Autodesk Fusion 360 part; units mm, degrees
(part 3 of 6)
sketch "top plate" plane through (0, 0, 0) normal (0, 1, 0) x (1, 0, 0)
  line L0 (103.8578, -14.9931) -> (9.2428, -14.9931)
  line L1 (9.2428, -110.3136) -> (21.2428, -111.7953)
  line L2 (21.2428, -111.7953) -> (66.9572, -117.4397)
  line L3 (66.9572, -117.4397) -> (84.9842, -117.4397)
  line L4 (123.6486, -112.6772) -> (84.9842, -117.4397)
  arc A0 (138.7122, -103.2228) -> (142.7339, -99.2011) centre (138.7122, -99.2011) ccw
  arc A1 (146.7556, -80.8214) -> (142.7339, -84.843) centre (146.7556, -84.843) ccw
  arc A2 (146.7556, -80.8214) -> (146.7556, -72.7781) centre (146.7556, -76.7997) ccw
  arc A3 (142.7339, -68.7564) -> (146.7556, -72.7781) centre (146.7556, -68.7564) ccw
  arc A4 (146.8111, -48.4919) -> (142.7339, -52.5692) centre (146.8111, -52.5692) ccw
  arc A5 (157.6917, -48.4919) -> (157.6917, -40.3375) centre (157.6917, -44.4147) ccw
  arc A6 (150.7772, -36.2632) -> (154.8573, -40.3375) centre (154.8544, -36.2603) ccw
  line L5 (142.6281, 7.5847) -> (103.8578, -14.9931)
  line L6 (142.6281, 7.5847) -> (161.7839, -25.5411)
  line L7 (132.0216, -103.2228) -> (138.7122, -103.2228)
  line L8 (142.7339, -99.2011) -> (142.7339, -84.843)
  line L9 (142.7339, -52.5692) -> (142.7339, -68.7564)
  line L10 (146.8111, -48.4919) -> (157.6917, -48.4919)
  line L11 (157.6917, -40.3375) -> (154.8573, -40.3375)
  line L12 (9.2428, -110.3136) -> (9.2428, -14.9931)
  line L13 (11.8031, -107.7533) -> (25.8031, -107.7533)
  line L14 (25.8031, -107.7533) -> (25.8031, -93.7533)
  line L15 (25.8031, -93.7533) -> (11.8031, -93.7533)
  line L16 (11.8031, -93.7533) -> (11.8031, -107.7533)
  line L17 (30.8531, -107.7533) -> (44.8531, -107.7533)
  line L18 (44.8531, -107.7533) -> (44.8531, -93.7533)
  line L19 (44.8531, -93.7533) -> (30.8531, -93.7533)
  line L20 (30.8531, -93.7533) -> (30.8531, -107.7533)
  line L21 (49.9031, -112.5158) -> (63.9031, -112.5158)
  line L22 (63.9031, -112.5158) -> (63.9031, -98.5158)
  line L23 (63.9031, -98.5158) -> (49.9031, -98.5158)
  line L24 (49.9031, -98.5158) -> (49.9031, -112.5158)
  line L25 (88.0031, -112.5158) -> (102.0031, -112.5158)
  line L26 (102.0031, -112.5158) -> (102.0031, -98.5158)
  line L27 (102.0031, -98.5158) -> (88.0031, -98.5158)
  line L28 (107.0531, -110.1169) -> (121.0531, -110.1169)
  line L29 (121.0531, -110.1169) -> (121.0531, -96.1169)
  line L30 (121.0531, -96.1169) -> (107.0531, -96.1169)
  line L31 (107.0531, -96.1169) -> (107.0531, -110.1169)
  line L32 (140.1031, -100.5919) -> (126.1031, -100.5919)
  line L33 (126.1031, -100.5919) -> (126.1031, -86.5919)
  line L34 (126.1031, -86.5919) -> (140.1031, -86.5919)
  line L35 (140.1031, -86.5919) -> (140.1031, -100.5919)
  line L36 (126.1031, -81.5419) -> (140.1031, -81.5419)
  line L37 (140.1031, -81.5419) -> (140.1031, -67.5419)
  line L38 (140.1031, -67.5419) -> (126.1031, -67.5419)
  line L39 (126.1031, -67.5419) -> (126.1031, -81.5419)
  line L40 (126.1031, -62.4919) -> (140.1031, -62.4919)
  line L41 (140.1031, -62.4919) -> (140.1031, -48.4919)
  line L42 (140.1031, -48.4919) -> (126.1031, -48.4919)
  line L43 (126.1031, -48.4919) -> (126.1031, -62.4919)
  line L44 (49.9031, -93.4658) -> (63.9031, -93.4658)
  line L45 (63.9031, -93.4658) -> (63.9031, -79.4658)
  line L46 (63.9031, -79.4658) -> (49.9031, -79.4658)
  line L47 (49.9031, -79.4658) -> (49.9031, -93.4658)
  line L48 (49.9031, -74.4158) -> (63.9031, -74.4158)
  line L49 (63.9031, -74.4158) -> (63.9031, -60.4158)
  line L50 (63.9031, -60.4158) -> (49.9031, -60.4158)
  line L51 (49.9031, -60.4158) -> (49.9031, -74.4158)
  line L52 (49.9031, -55.3658) -> (63.9031, -55.3658)
  line L53 (63.9031, -55.3658) -> (63.9031, -41.3658)
  line L54 (63.9031, -41.3658) -> (49.9031, -41.3658)
  line L55 (49.9031, -41.3658) -> (49.9031, -55.3658)
  line L56 (30.8531, -88.7033) -> (44.8531, -88.7033)
  line L57 (44.8531, -88.7033) -> (44.8531, -74.7033)
  line L58 (44.8531, -74.7033) -> (30.8531, -74.7033)
  line L59 (30.8531, -74.7033) -> (30.8531, -88.7033)
  line L60 (30.8531, -69.6533) -> (44.8531, -69.6533)
  line L61 (44.8531, -69.6533) -> (44.8531, -55.6533)
  line L62 (44.8531, -55.6533) -> (30.8531, -55.6533)
  line L63 (30.8531, -55.6533) -> (30.8531, -69.6533)
  line L64 (11.8031, -88.7033) -> (25.8031, -88.7033)
  line L65 (25.8031, -88.7033) -> (25.8031, -74.7033)
  line L66 (25.8031, -74.7033) -> (11.8031, -74.7033)
  line L67 (11.8031, -74.7033) -> (11.8031, -88.7033)
  line L68 (11.8031, -69.6533) -> (25.8031, -69.6533)
  line L69 (25.8031, -69.6533) -> (25.8031, -55.6533)
  line L70 (25.8031, -55.6533) -> (11.8031, -55.6533)
  line L71 (11.8031, -55.6533) -> (11.8031, -69.6533)
  line L72 (11.8031, -50.6033) -> (25.8031, -50.6033)
  line L73 (25.8031, -50.6033) -> (25.8031, -36.6033)
  line L74 (25.8031, -36.6033) -> (11.8031, -36.6033)
  line L75 (11.8031, -36.6033) -> (11.8031, -50.6033)
  line L76 (30.8531, -50.6033) -> (44.8531, -50.6033)
  line L77 (44.8531, -50.6033) -> (44.8531, -36.6033)
  line L78 (44.8531, -36.6033) -> (30.8531, -36.6033)
  line L79 (30.8531, -36.6033) -> (30.8531, -50.6033)
  line L80 (11.8031, -31.5533) -> (25.8031, -31.5533)
  line L81 (25.8031, -31.5533) -> (25.8031, -17.5533)
  line L82 (25.8031, -17.5533) -> (11.8031, -17.5533)
  line L83 (11.8031, -17.5533) -> (11.8031, -31.5533)
  line L84 (30.8531, -31.5533) -> (44.8531, -31.5533)
  line L85 (44.8531, -31.5533) -> (44.8531, -17.5533)
  line L86 (44.8531, -17.5533) -> (30.8531, -17.5533)
  line L87 (30.8531, -17.5533) -> (30.8531, -31.5533)
  line L88 (49.9031, -36.3158) -> (63.9031, -36.3158)
  line L89 (63.9031, -36.3158) -> (63.9031, -22.3158)
  line L90 (63.9031, -22.3158) -> (49.9031, -22.3158)
  line L91 (49.9031, -22.3158) -> (49.9031, -36.3158)
  line L92 (68.9531, -114.8794) -> (82.9531, -114.8794)
  line L93 (82.9531, -114.8794) -> (82.9531, -100.8794)
  line L94 (82.9531, -100.8794) -> (68.9531, -100.8794)
  line L95 (68.9531, -100.8794) -> (68.9531, -114.8794)
  line L96 (68.9531, -95.8294) -> (82.9531, -95.8294)
  line L97 (82.9531, -95.8294) -> (82.9531, -81.8294)
  line L98 (82.9531, -81.8294) -> (68.9531, -81.8294)
  line L99 (68.9531, -81.8294) -> (68.9531, -95.8294)
  line L100 (68.9531, -76.7794) -> (82.9531, -76.7794)
  line L101 (82.9531, -76.7794) -> (82.9531, -62.7794)
  line L102 (82.9531, -62.7794) -> (68.9531, -62.7794)
  line L103 (68.9531, -62.7794) -> (68.9531, -76.7794)
  line L104 (68.9531, -57.7294) -> (82.9531, -57.7294)
  line L105 (82.9531, -57.7294) -> (82.9531, -43.7294)
  line L106 (82.9531, -43.7294) -> (68.9531, -43.7294)
  line L107 (68.9531, -43.7294) -> (68.9531, -57.7294)
  line L108 (76.5731, -36.3158) -> (90.5731, -36.3158)
  line L109 (90.5731, -36.3158) -> (90.5731, -22.3158)
  line L110 (90.5731, -22.3158) -> (76.5731, -22.3158)
  line L111 (76.5731, -22.3158) -> (76.5731, -36.3158)
  line L112 (88.0031, -74.4158) -> (102.0031, -74.4158)
  line L113 (102.0031, -74.4158) -> (102.0031, -60.4158)
  line L114 (102.0031, -60.4158) -> (88.0031, -60.4158)
  line L115 (88.0031, -60.4158) -> (88.0031, -74.4158)
  line L116 (107.0531, -77.0669) -> (121.0531, -77.0669)
  line L117 (121.0531, -77.0669) -> (121.0531, -91.0669)
  line L118 (121.0531, -91.0669) -> (107.0531, -91.0669)
  line L119 (107.0531, -91.0669) -> (107.0531, -77.0669)
  line L120 (88.0031, -93.4658) -> (102.0031, -93.4658)
  line L121 (102.0031, -93.4658) -> (102.0031, -79.4658)
  line L122 (102.0031, -79.4658) -> (88.0031, -79.4658)
  line L123 (88.0031, -79.4658) -> (88.0031, -93.4658)
  line L124 (107.0531, -72.0169) -> (121.0531, -72.0169)
  line L125 (121.0531, -72.0169) -> (121.0531, -58.0169)
  line L126 (121.0531, -58.0169) -> (107.0531, -58.0169)
  line L127 (107.0531, -58.0169) -> (107.0531, -72.0169)
  line L128 (107.0531, -52.9669) -> (121.0531, -52.9669)
  line L129 (121.0531, -52.9669) -> (121.0531, -38.9669)
  line L130 (121.0531, -38.9669) -> (107.0531, -38.9669)
  line L131 (107.0531, -38.9669) -> (107.0531, -52.9669)
  line L132 (88.0031, -55.3658) -> (102.0031, -55.3658)
  line L133 (102.0031, -55.3658) -> (102.0031, -41.3658)
  line L134 (102.0031, -41.3658) -> (88.0031, -41.3658)
  line L135 (88.0031, -41.3658) -> (88.0031, -55.3658)
  line L136 (88.0031, -112.5158) -> (88.0031, -98.5158)
  circle A7 centre (28.3281, -91.2283) radius 1.1
  circle A8 centre (18.8031, -34.0783) radius 1.1
  circle A9 centre (71.0494, -18.8031) radius 1.1
  circle A10 centre (95.25, -34.2547) radius 1.1
  circle A11 centre (115.7464, -33.7256) radius 1.1
  circle A12 centre (146.7556, -76.7997) radius 1.1
  circle A13 centre (157.6917, -44.4147) radius 1.1
  circle A14 centre (146.7556, -37.8883) radius 1.1
  circle A15 centre (123.5781, -102.5878) radius 1.1
  circle A16 centre (66.4281, -78.105) radius 1.1
  circle A17 centre (130.9158, -10.2658) radius 1.1
  line L137 (104.7731, -17.2287) -> (111.7731, -29.353)
  line L138 (111.7731, -29.353) -> (123.8975, -22.353)
  line L139 (123.8975, -22.353) -> (116.8975, -10.2287)
  line L140 (116.8975, -10.2287) -> (104.7731, -17.2287)
  line L141 (139.0984, -19.4159) -> (146.0984, -31.5402)
  line L142 (146.0984, -31.5402) -> (158.2227, -24.5402)
  line L143 (158.2227, -24.5402) -> (151.2227, -12.4159)
  line L144 (151.2227, -12.4159) -> (139.0984, -19.4159)
  line L145 (161.7839, -25.5411) -> (150.0604, -32.3205)
  line L146 (154.8544, -36.2603) -> (154.8544, -34.2581)
  line L147 (150.7772, -36.2632) -> (150.7772, -32.2)
  line L148 (154.8544, -34.2581) -> (152.8134, -30.7285)
  arc A18 (152.8134, -30.7285) -> (150.7772, -34.2581) centre (154.8544, -34.2581) ccw
  line L149 (122.5884, -28.9762) -> (129.5884, -41.1005)
  line L150 (129.5884, -41.1005) -> (141.7127, -34.1005)
  line L151 (141.7127, -34.1005) -> (134.7127, -21.9762)
  line L152 (134.7127, -21.9762) -> (122.5884, -28.9762)
  line L153 (129.5734, -2.9059) -> (136.5734, -15.0302)
  line L154 (136.5734, -15.0302) -> (148.6977, -8.0302)
  line L155 (148.6977, -8.0302) -> (141.6977, 4.0941)
  line L156 (141.6977, 4.0941) -> (129.5734, -2.9059)
  line L157 (123.6486, -112.6772) -> (123.6486, -108.4548)
  line L158 (123.6486, -108.4548) -> (127.6703, -108.4548)
  arc A19 (126.6957, -104.553) -> (123.6486, -108.4548) centre (127.6703, -108.4548) ccw
  line L159 (132.0216, -103.2228) -> (126.6957, -104.553)
  line L160 (127.6703, -108.4548) -> (126.6957, -104.553)
  line L161 (161.7839, -103.1522) -> (123.6486, -112.6772)
  line L162 (103.943, -25.7908) -> (124.7276, -13.7908)
  line L163 (98.3098, -21.884) -> (104.5098, -32.6227)
  line L164 (104.5098, -32.6227) -> (109.5761, -29.6977)
  line L165 (109.5761, -29.6977) -> (103.3761, -18.959)
  line L166 (103.3761, -18.959) -> (98.3098, -21.884)
  line L167 (124.1607, -6.959) -> (130.3607, -17.6977)
  line L168 (130.3607, -17.6977) -> (125.2945, -20.6227)
  line L169 (125.2945, -20.6227) -> (119.0945, -9.884)
  line L170 (119.0945, -9.884) -> (124.1607, -6.959)
  line L171 (107.9761, -26.9264) -> (109.7731, -25.8889)
  line L172 (104.9761, -21.7303) -> (106.7731, -20.6928)
  line L173 (121.8975, -18.8889) -> (123.6945, -17.8514)
  line L174 (118.8975, -13.6928) -> (120.6945, -12.6553)
  line L175 (131.5417, -103.3426) -> (132.5162, -107.2444)
  line L176 (132.5162, -103.2228) -> (132.5162, -107.2444)
  arc A20 (132.5162, -103.2228) -> (131.5417, -103.3426) centre (132.5162, -107.2444) ccw
  point P0 (132.0216, -103.2228)
  point P1 (18.8031, -100.7533)
  point P2 (37.8531, -100.7533)
  point P3 (37.8531, -81.7033)
  point P4 (28.3281, -91.2283)
  point P5 (18.8031, -81.7033)
  point P6 (56.9031, -105.5158)
  point P7 (56.9031, -86.4658)
  point P8 (18.8031, -62.6533)
  point P9 (37.8531, -62.6533)
  point P10 (56.9031, -67.4158)
  point P11 (56.9031, -48.3658)
  point P12 (37.8531, -43.6033)
  point P13 (18.8031, -43.6033)
  point P14 (18.8031, -24.5533)
  point P15 (18.8031, -34.0783)
  point P16 (37.8531, -24.5533)
  point P17 (56.9031, -29.3158)
  point P18 (71.0494, -18.8031)
  point P19 (83.5731, -29.3158)
  point P20 (95.25, -34.2547)
  point P21 (115.7464, -33.7256)
  point P22 (114.3353, -19.7908)
  point P23 (132.1506, -31.5383)
  point P24 (130.9158, -10.2658)
  point P25 (139.1356, -5.4681)
  point P26 (148.6606, -21.9781)
  point P27 (146.7556, -37.8883)
  point P28 (157.6917, -44.4147)
  point P29 (114.0531, -45.9669)
  point P30 (133.1031, -55.4919)
  point P31 (114.0531, -65.0169)
  point P32 (95.0031, -48.3658)
  point P33 (95.0031, -67.4158)
  point P34 (133.1031, -74.5419)
  point P35 (146.7556, -76.7997)
  point P36 (133.1031, -93.5919)
  point P37 (123.5781, -102.5878)
  point P38 (114.0531, -103.1169)
  point P39 (114.0531, -84.0669)
  point P40 (95.0031, -86.4658)
  point P41 (95.0031, -105.5158)
  point P42 (66.4281, -78.105)
  point P43 (75.9531, -107.8794)
  point P44 (75.9531, -88.8294)
  point P45 (75.9531, -69.7794)
  point P46 (75.9531, -50.7294)
  dimension "d126" = 14
  dimension "d127" = 14
  dimension "d128" = 7
  dimension "d129" = 7
  dimension "d130" = 14
  dimension "d131" = 14
  dimension "d132" = 14
  dimension "d133" = 14
  dimension "d134" = 14
  dimension "d135" = 14
  dimension "d136" = 14
  dimension "d137" = 14
  dimension "d138" = 14
  dimension "d139" = 14
  dimension "d140" = 14
  dimension "d141" = 14
  dimension "d142" = 14
  dimension "d143" = 14
  dimension "d144" = 14
  dimension "d145" = 14
  dimension "d146" = 14
  dimension "d147" = 14
  dimension "d148" = 14
  dimension "d149" = 14
  dimension "d150" = 14
  dimension "d151" = 14
  dimension "d152" = 14
  dimension "d153" = 14
  dimension "d154" = 14
  dimension "d155" = 14
  dimension "d156" = 14
  dimension "d157" = 14
  dimension "d158" = 14
  dimension "d159" = 14
  dimension "d160" = 14
  dimension "d161" = 14
  dimension "d162" = 14
  dimension "d163" = 14
  dimension "d164" = 14
  dimension "d165" = 14
  dimension "d166" = 14
  dimension "d167" = 14
  dimension "d168" = 14
  dimension "d170" = 14
  dimension "d171" = 14
  dimension "d172" = 14
  dimension "d173" = 14
  dimension "d174" = 14
  dimension "d175" = 14
  dimension "d176" = 14
  dimension "d177" = 14
  dimension "d178" = 14
  dimension "d179" = 14
  dimension "d180" = 14
  dimension "d181" = 14
  dimension "d182" = 14
  dimension "d183" = 14
  dimension "d184" = 14
  dimension "d185" = 14
  dimension "d186" = 14
  dimension "d187" = 14
  dimension "d188" = 14
  dimension "d189" = 14
  dimension "d190" = 7
  dimension "d191" = 7
  dimension "d192" = 7
  dimension "d193" = 7
  dimension "d194" = 7
  dimension "d195" = 7
  dimension "d196" = 7
  dimension "d197" = 7
  dimension "d198" = 7
  dimension "d199" = 7
  dimension "d200" = 7
  dimension "d201" = 7
  dimension "d202" = 14
  dimension "d203" = 7
  dimension "d204" = 7
  dimension "d205" = 7
  dimension "d206" = 7
  dimension "d207" = 7
  dimension "d208" = 7
  dimension "d209" = 7
  dimension "d210" = 7
  dimension "d211" = 7
  dimension "d212" = 7
  dimension "d213" = 7
  dimension "d214" = 7
  dimension "d215" = 7
  dimension "d216" = 7
  dimension "d217" = 7
  dimension "d218" = 7
  dimension "d219" = 7
  dimension "d220" = 7
  dimension "d221" = 7
  dimension "d222" = 7
  dimension "d223" = 7
  dimension "d224" = 7
  dimension "d225" = 7
  dimension "d226" = 7
  dimension "d227" = 7
  dimension "d228" = 7
  dimension "d229" = 7
  dimension "d230" = 7
  dimension "d231" = 7
  dimension "d232" = 7
  dimension "d233" = 7
  dimension "d234" = 7
  dimension "d235" = 7
  dimension "d236" = 7
  dimension "d237" = 7
  dimension "d238" = 7
  dimension "d239" = 7
  dimension "d240" = 7
  dimension "d241" = 7
  dimension "d242" = 7
  dimension "d243" = 7
  dimension "d244" = 7
  dimension "d245" = 7
  dimension "d246" = 7
  dimension "d247" = 7
  dimension "d248" = 7
  dimension "d249" = 7
  dimension "d250" = 7
  dimension "d251" = 2.2
  dimension "d252" = 2.2
  dimension "d253" = 2.2
  dimension "d254" = 2.2
  dimension "d255" = 2.2
  dimension "d256" = 2.2
  dimension "d257" = 2.2
  dimension "d258" = 2.2
  dimension "d259" = 2.2
  dimension "d260" = 2.2
  dimension "d261" = 2.2
  dimension "d262" = 14
  dimension "d263" = 14
  dimension "d264" = 150
  dimension "d265" = 7
  dimension "d266" = 7
  dimension "d267" = 14
  dimension "d268" = 14
  dimension "d269" = 7
  dimension "d270" = 7
  dimension "d271" = 4.0772
  dimension "d272" = 4.0772
  dimension "d273" = 14
  dimension "d274" = 14
  dimension "d275" = 7
  dimension "d276" = 7
  dimension "d277" = 14
  dimension "d278" = 14
  dimension "d279" = 7
  dimension "d280" = 7
  dimension "d281" = 4.0217
  dimension "d282" = 4.0217
  dimension "d284" = 24
  dimension "d285" = 5.85
  dimension "d286" = 2.925
  dimension "d287" = 12
  dimension "d288" = 5.85
  dimension "d289" = 2.925
  dimension "d290" = 12.4
  dimension "d291" = 6.2
  dimension "d292" = 12.4
  dimension "d293" = 6.2
  dimension "d294" = 6
  dimension "d295" = 6
  dimension "d296" = 3
  dimension "d297" = 3
  dimension "d298" = 4.0217
  dimension "d299" = 4.0217
  constraint coincident P0 L7.start
  constraint coincident A0.start L7.end
  constraint coincident A0.end L8.start
  constraint coincident A1.end L8.end
  constraint coincident A4.end L9.start
  constraint coincident A3.start L9.end
  constraint coincident A4.start L10.start
  constraint coincident A5.start L10.end
  constraint coincident A5.end L11.start
  constraint coincident A6.end L11.end
  constraint coincident L1.start L12.start
  constraint coincident L0.end L12.end
  constraint horizontal L13
  constraint vertical L14
  constraint horizontal L15
  constraint vertical L16
  constraint horizontal L17
  constraint vertical L18
  constraint horizontal L19
  constraint vertical L20
  constraint horizontal L21
  constraint vertical L22
  constraint horizontal L23
  constraint vertical L24
  constraint horizontal L25
  constraint vertical L26
  constraint horizontal L27
  constraint horizontal L28
  constraint vertical L29
  constraint horizontal L30
  constraint vertical L31
  constraint horizontal L32
  constraint vertical L33
  constraint horizontal L34
  constraint vertical L35
  constraint horizontal L36
  constraint vertical L37
  constraint horizontal L38
  constraint vertical L39
  constraint horizontal L40
  constraint vertical L41
  constraint horizontal L42
  constraint vertical L43
  constraint horizontal L44
  constraint vertical L45
  constraint horizontal L46
  constraint vertical L47
  constraint horizontal L48
  constraint vertical L49
  constraint horizontal L50
  constraint vertical L51
  constraint horizontal L52
  constraint vertical L53
  constraint horizontal L54
  constraint vertical L55
  constraint horizontal L56
  constraint vertical L57
  constraint horizontal L58
  constraint vertical L59
  constraint horizontal L60
  constraint vertical L61
  constraint horizontal L62
  constraint vertical L63
  constraint horizontal L64
  constraint vertical L65
  constraint horizontal L66
  constraint vertical L67
  constraint horizontal L68
  constraint vertical L69
  constraint horizontal L70
  constraint vertical L71
  constraint horizontal L72
  constraint vertical L73
  constraint horizontal L74
  constraint vertical L75
  constraint horizontal L76
  constraint vertical L77
  constraint horizontal L78
  constraint vertical L79
  constraint horizontal L80
  constraint vertical L81
  constraint horizontal L82
  constraint vertical L83
  constraint horizontal L84
  constraint vertical L85
  constraint horizontal L86
  constraint vertical L87
  constraint horizontal L88
  constraint vertical L89
  constraint horizontal L90
  constraint vertical L91
  constraint horizontal L92
  constraint vertical L93
  constraint horizontal L94
  constraint vertical L95
  constraint horizontal L96
  constraint vertical L97
  constraint horizontal L98
  constraint vertical L99
  constraint horizontal L100
  constraint vertical L101
  constraint horizontal L102
  constraint vertical L103
  constraint horizontal L104
  constraint vertical L105
  constraint horizontal L106
  constraint vertical L107
  constraint horizontal L108
  constraint vertical L109
  constraint horizontal L110
  constraint vertical L111
  constraint horizontal L112
  constraint vertical L113
  constraint horizontal L114
  constraint vertical L115
  constraint horizontal L116
  constraint vertical L117
  constraint horizontal L118
  constraint vertical L119
  constraint horizontal L120
  constraint vertical L121
  constraint horizontal L122
  constraint vertical L123
  constraint horizontal L124
  constraint vertical L125
  constraint horizontal L126
  constraint vertical L127
  constraint horizontal L128
  constraint vertical L129
  constraint horizontal L130
  constraint vertical L131
  constraint horizontal L132
  constraint vertical L133
  constraint horizontal L134
  constraint vertical L135
  constraint perpendicular L25 L136
  constraint coincident P4 A7.centre
  constraint coincident P15 A8.centre
  constraint coincident P18 A9.centre
  constraint coincident P20 A10.centre
  constraint coincident P21 A11.centre
  constraint concentric A2 A12
  constraint concentric A5 A13
  constraint coincident P27 A14.centre
  constraint coincident P37 A15.centre
  constraint coincident P42 A16.centre
  constraint coincident P24 A17.centre
  constraint perpendicular L138 L139
  constraint perpendicular L137 L138
  constraint perpendicular L137 L140
  constraint parallel L141 L143
  constraint perpendicular L141 L144
  constraint perpendicular L142 L143
  constraint parallel L138 L144
  constraint coincident L6.end L145.start
  constraint perpendicular L6 L145
  constraint coincident A6.centre L146.start
  constraint vertical L146
  constraint coincident A6.start L147.start
  constraint vertical L147
  constraint coincident L145 L148.end
  constraint perpendicular L145 L148
  constraint coincident L148 A18.start
  constraint coincident L147 A18.end
  constraint coincident L146.end L148.start
  constraint perpendicular L149 L150
  constraint perpendicular L151 L152
  constraint parallel L149 L151
  constraint parallel L138 L152
  constraint perpendicular L153 L156
  constraint perpendicular L154 L155
  constraint parallel L153 L155
  constraint parallel L140 L156
  constraint coincident L4.start L157.start
  constraint parallel L29 L157
  constraint perpendicular L157 L158
  constraint coincident L158.end A19.centre
  constraint coincident L159 A19.start
  constraint perpendicular L159 L160
  constraint coincident A19.start L159.end
  constraint parallel L159 L161
  constraint perpendicular L168 L169
  constraint coincident P22 L162
  constraint perpendicular L163 L166
  constraint perpendicular L164 L165
  constraint parallel L163 L165
  constraint perpendicular L167 L170
  constraint parallel L167 L169
  constraint parallel L138 L162
  constraint parallel L162 L164
  constraint parallel L162 L168
  constraint coincident L165 L171.start
  constraint coincident L137 L171.end
  constraint perpendicular L137 L171
  constraint coincident L165 L172.start
  constraint coincident L137 L172.end
  constraint perpendicular L137 L172
  constraint coincident L139 L173.start
  constraint coincident L169 L173.end
  constraint perpendicular L169 L173
  constraint coincident L139 L174.start
  constraint coincident L169 L174.end
  constraint perpendicular L169 L174
  constraint coincident L159 L175.start
  constraint perpendicular L159 L175
  constraint coincident L7 L176.start
  constraint perpendicular L7 L176
  constraint coincident L175.end L176.end
  measures "d126" distance of L13.start L13.end
  measures "d127" distance of L13.start L15.end
  measures "d128" distance of P1 L16
  measures "d129" distance of P1 L15
  measures "d130" distance of L80.start L80.end
  measures "d131" distance of L80.start L82.end
  measures "d132" distance of L108.start L108.end
  measures "d133" distance of L108.start L110.end
  measures "d134" distance of L17.start L17.end
  measures "d135" distance of L17.start L19.end
  measures "d136" distance of L21.start L23.end
  measures "d137" distance of L21.start L21.end
  measures "d138" distance of L44.start L44.end
  measures "d139" distance of L44.start L46.end
  measures "d140" distance of L56.start L56.end
  measures "d141" distance of L56.start L58.end
  measures "d142" distance of L64.start L66.end
  measures "d143" distance of L64.start L64.end
  measures "d144" distance of L68.start L68.end
  measures "d145" distance of L68.start L70.end
  measures "d146" distance of L72.start L74.end
  measures "d147" distance of L72.start L72.end
  measures "d148" distance of L84.start L86.end
  measures "d149" distance of L84.start L84.end
  measures "d150" distance of L76.start L78.end
  measures "d151" distance of L76.start L76.end
  measures "d152" distance of L60.start L62.end
  measures "d153" distance of L60.start L60.end
  measures "d154" distance of L48.start L50.end
  measures "d155" distance of L48.start L48.end
  measures "d156" distance of L52.start L54.end
  measures "d157" distance of L52.start L52.end
  measures "d158" distance of L88.start L88.end
  measures "d159" distance of L88.start L90.end
  measures "d160" distance of L104.start L106.end
  measures "d161" distance of L104.start L104.end
  measures "d162" distance of L100.start L102.end
  measures "d163" distance of L100.start L100.end
  measures "d164" distance of L96.start L98.end
  measures "d165" distance of L96.start L96.end
  measures "d166" distance of L92.start L92.end
  measures "d167" distance of L92.start L94.end
  measures "d168" distance of L25.end L26.end
  measures "d170" distance of L120.start L120.end
  measures "d171" distance of L120.start L122.end
  measures "d172" distance of L117.end L118.end
  measures "d173" distance of L28.start L30.end
  measures "d174" distance of L28.start L28.end
  measures "d175" distance of L33.end L34.end
  measures "d176" distance of L32.end L33.end
  measures "d177" distance of L116.start L118.end
  measures "d178" distance of L36.start L38.end
  measures "d179" distance of L36.start L36.end
  measures "d180" distance of L124.start L124.end
  measures "d181" distance of L124.start L126.end
  measures "d182" distance of L112.start L112.end
  measures "d183" distance of L112.start L114.end
  measures "d184" distance of L132.start L132.end
  measures "d185" distance of L132.start L134.end
  measures "d186" distance of L128.start L130.end
  measures "d187" distance of L128.start L128.end
  measures "d188" distance of L40.start L42.end
  measures "d189" distance of L41.end L42.end
  measures "d190" distance of P2 L20
  measures "d191" distance of P2 L17
  measures "d192" distance of P5 L64
  measures "d193" distance of P5 L67
  measures "d194" distance of P3 L56
  measures "d195" distance of P3 L59
  measures "d196" distance of P7 L47
  measures "d197" distance of P7 L44
  measures "d198" distance of P6 L24
  measures "d199" distance of P6 L21
  measures "d200" distance of P43 L92
  measures "d201" distance of P43 L95
  measures "d202" distance of L25.start L25.end
  measures "d203" distance of P41 L136
  measures "d204" distance of P41 L25
  measures "d205" distance of P38 L28
  measures "d206" distance of P38 L31
  measures "d207" distance of P36 L32
  measures "d208" distance of P36 L33
  measures "d209" distance of P34 L36
  measures "d210" distance of P34 L39
  measures "d211" distance of P30 L40
  measures "d212" distance of P30 L43
  measures "d213" distance of P29 L128
  measures "d214" distance of P29 L131
  measures "d215" distance of P31 L124
  measures "d216" distance of P31 L127
  measures "d217" distance of P39 L117
  measures "d218" distance of P39 L116
  measures "d219" distance of P33 L113
  measures "d220" distance of P33 L112
  measures "d221" distance of P40 L121
  measures "d222" distance of P40 L122
  measures "d223" distance of P32 L133
  measures "d224" distance of P32 L134
  measures "d225" distance of P46 L104
  measures "d226" distance of P46 L107
  measures "d227" distance of P45 L100
  measures "d228" distance of P45 L103
  measures "d229" distance of P44 L97
  measures "d230" distance of P44 L98
  measures "d231" distance of P10 L49
  measures "d232" distance of P10 L48
  measures "d233" distance of P9 L60
  measures "d234" distance of P9 L63
  measures "d235" distance of P8 L69
  measures "d236" distance of P8 L68
  measures "d237" distance of P13 L72
  measures "d238" distance of P13 L75
  measures "d239" distance of P12 L79
  measures "d240" distance of P12 L76
  measures "d241" distance of P11 L55
  measures "d242" distance of P11 L52
  measures "d243" distance of P14 L80
  measures "d244" distance of P14 L83
  measures "d245" distance of P16 L84
  measures "d246" distance of P16 L87
  measures "d247" distance of P17 L88
  measures "d248" distance of P17 L91
  measures "d249" distance of P19 L108
  measures "d250" distance of P19 L111
  measures "d251" diameter of A7
  measures "d252" diameter of A8
  measures "d253" diameter of A9
  measures "d254" diameter of A10
  measures "d255" diameter of A11
  measures "d256" diameter of A12
  measures "d257" diameter of A13
  measures "d258" diameter of A14
  measures "d259" diameter of A15
  measures "d260" diameter of A16
  measures "d261" diameter of A17
  measures "d262" distance of L137.start L139.end
  measures "d263" distance of L138 L140
  measures "d264" angle of L110 L140
  measures "d265" distance of P22 L140
  measures "d266" distance of P22 L137
  measures "d267" distance of L142 L144
  measures "d268" distance of L141 L143
  measures "d269" distance of P26 L141
  measures "d270" distance of P26 L142
  measures "d271" horizontal distance of A6.start A6.centre
  measures "d272" distance of L146.end L148.end
  measures "d273" distance of L149.start L149.end
  measures "d274" distance of L149 L151
  measures "d275" distance of P23 L149
  measures "d276" distance of P23 L152
  measures "d277" distance of L153.start L153.end
  measures "d278" distance of L153.start L155.end
  measures "d279" distance of P25 L153
  measures "d280" distance of P25 L156
  measures "d281" radius of A0
  measures "d282" radius of A19
  measures "d284" distance of L162.start L162.end
  measures "d285" distance of L163.end L164.end
  measures "d286" distance of L162.start L165
  measures "d287" distance of P22 L162.start
  measures "d288" distance of L167.end L168.end
  measures "d289" distance of L162.end L169
  measures "d290" distance of L168.end L169.end
  measures "d291" distance of L162 L170
  measures "d292" distance of L163.start L163.end
  measures "d293" distance of L162.start L166
  measures "d294" distance of L173 L174
  measures "d295" distance of L171 L172
  measures "d296" distance of L162 L173
  measures "d297" distance of L162 L172
  measures "d298" distance of L175.start L175.end
  measures "d299" distance of L176.start L175.end
extrude "Extrude1" add sketch "top plate" along normal blind 1.2 contours L0 L1 L2 L3 L4 A0 A1 A2 A3 A4 A5 A6 L5 L6 L7 L8 L9 L10 L11 L12 L145 L147 A18 L157 A19 L159 | L7 L159 A20 makes body 1
extrude "Extrude2" add sketch "PCB" along normal blind 1.2 from surface at 2.5 separate body makes body 2
sketch "nn adapter" plane through (0, 3.7, 0) normal (0, 1, 0) x (-1, 0, 0)
  line L0 (-142.6281, -7.5847) -> (-103.8578, 14.9931)
  line L1 (-103.8578, 14.9931) -> (-9.2428, 14.9931)
  line L2 (-9.2428, 14.9931) -> (-9.2428, 110.3136)
  line L3 (-9.2428, 110.3136) -> (-66.9572, 117.4397)
  line L4 (-66.9572, 117.4397) -> (-84.9842, 117.4397)
  line L5 (-84.9842, 117.4397) -> (-123.6486, 112.6772)
  line L6 (-123.6486, 112.6772) -> (-161.7839, 103.1522)
  line L7 (-161.7839, 103.1522) -> (-161.7839, 25.5411)
  line L8 (-161.7839, 25.5411) -> (-142.6281, -7.5847)
  line L9 (-63.7469, 114.0531) -> (-63.7469, 81.6681)
  line L10 (-86.36, 81.6328) -> (-86.36, 114.0531)
  line L11 (-86.36, 114.0531) -> (-63.7469, 114.0531)
  line L12 (-63.7469, 81.6681) -> (-86.36, 81.6328)
  constraint coincident L10.end L11.start
  constraint coincident L9.start L11.end
  constraint coincident L9.end L12.start
  constraint coincident L10.start L12.end
extrude "Extrude3" add sketch "nn adapter" along normal blind 1.2 from surface at 2.413 separate body contours L9 L10 L11 L12 makes body 3
ref_plane "WorkPlane1" through (85.5133, 6.2, 54.9275) normal (0, 1, 0) x (1, 0, 0)
extrude "Extrude4" add sketch "baseplate" along normal blind 5.6 from surface at 6.2 separate body makes body 4
ref_plane "WorkPlane2" through (85.5133, 5.55, 54.9275) normal (0, 1, 0) x (0, 0, 1)
sketch "battery" plane through (85.5133, 5.55, 54.9275) normal (0, 1, 0) x (1, 0, 0)
  line L0 (57.75, -26.2553) -> (-57.75, -26.2553)
  line L1 (-57.75, -26.2553) -> (-57.75, 38.7447)
  line L2 (-57.75, 38.7447) -> (57.75, 38.7447)
  line L3 (57.75, 38.7447) -> (57.75, -26.2553)
  line L4 (-21.9664, -26.5053) -> (-54.2706, -26.5053)
  line L5 (58.2706, 38.9947) -> (58.2706, -30.5053)
  line L6 (-58.2706, 38.9947) -> (54.2706, 38.9947)
  line L7 (-58.2706, -26.5053) -> (-58.2706, 34.9947)
  dimension "d326" = 115.5
  dimension "d327" = 65
  dimension "d328" = 0.5206
  dimension "d329" = 0.5206
  dimension "d330" = 0.25
  dimension "d331" = 0.25
  constraint horizontal L0
  constraint vertical L1
  constraint horizontal L2
  constraint vertical L3
  measures "d326" distance of L0.start L0.end
  measures "d327" distance of L0.start L2.end
  measures "d328" distance of L3 L5
  measures "d329" distance of L1 L7
  measures "d330" distance of L0 L4
  measures "d331" distance of L2 L6
extrude "Extrude5" add sketch "battery" along normal blind 8.8 separate body makes body 5
sketch "mock nn" plane through (0, 7.313, 0) normal (0, 1, 0) x (-1, 0, 0)
  line L0 (-63.7469, 81.6681) -> (-63.7469, 114.0531)
  line L1 (-63.7469, 114.0531) -> (-86.36, 114.0531)
  line L2 (-86.36, 114.0531) -> (-86.36, 81.6328)
  line L3 (-86.36, 81.6328) -> (-63.7469, 81.6681)
extrude "Extrude6" add sketch "mock nn" along normal blind 1.2 from surface at 2.413 separate body makes body 6
extrude "Extrude7" add sketch "battery plate" along normal blind 1.6 from surface at 14.8 separate body makes body 7
ref_plane "WorkPlane4" through (85.5133, -9.7, 54.9275) normal (0, -1, 0) x (-1, 0, 0)